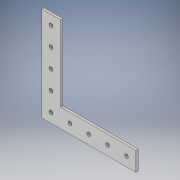
# Autodesk Inventor part: L gusset
Saved by Autodesk Inventor 2018 (Build 220112000, 112)
## iProperties
Created: 2019-01-13
Part Number: L gusset
Material: Generic
Document SubType Name: Modeling
Designer: s-2512711
Density: 1 g/cm^3
Appearance: Default
Author: s-2512711
Autodesk Inventor part; units mm, degrees
ref_plane "YZ Plane" through (0, 0, 0) normal (1, 0, 0) x (0, 1, 0)
ref_plane "XZ Plane" through (0, 0, 0) normal (0, 1, 0) x (-1, 0, 0)
ref_plane "XY Plane" through (0, 0, 0) normal (0, 0, 1) x (1, 0, 0)
sketch "Sketch1" plane through (0, 0, 0) normal (0, 0, 1) x (1, 0, 0)
  line L0 (0, 0) -> (76.2, 0)
  line L1 (76.2, 0) -> (76.2, 25.4)
  line L2 (76.2, 25.4) -> (25.4, 25.4)
  line L3 (0, 25.4) -> (0, 0)
  line L4 (0, 0) -> (25.4, 0)
  line L5 (25.4, 25.4) -> (25.4, 76.2)
  line L6 (25.4, 76.2) -> (0, 76.2)
  line L7 (0, 76.2) -> (0, 0)
  line L8 (12.7, 76.2) -> (12.7, 63.5) construction
  line L9 (12.7, 63.5) -> (12.7, 38.1) construction
  line L10 (12.7, 38.1) -> (12.7, 12.7) construction
  line L11 (12.7, 12.7) -> (38.1, 12.7) construction
  line L12 (38.1, 12.7) -> (63.5, 12.7) construction
  circle A0 centre (12.7, 63.5) radius 2.5797
  circle A1 centre (12.7, 38.1) radius 2.5797
  circle A2 centre (12.7, 12.7) radius 2.5797
  circle A3 centre (38.1, 12.7) radius 2.5797
  circle A4 centre (63.5, 12.7) radius 2.5797
  dimension "d0" = 76.2
  dimension "d1" = 25.4
  dimension "d2" = 25.4
  dimension "d3" = 76.2
  dimension "d4" = 12.7
  dimension "d5" = 25.4
  dimension "d6" = 25.4
  dimension "d7" = 25.4
  dimension "d8" = 25.4
  dimension "d9" = 5.1594
  constraints: 26 end point, 5 centre point, 5 coincident, 4 parallel, 3 perpendicular, 3 point on line, 2 horizontal, 1 midpoint, 1 vertical
  measures "d0" distance of L3.start L1.end
  measures "d1" distance of L1.end L0.end
  measures "d2" distance of L6.end L5.end
  measures "d3" distance of L5.end L4.end
  measures "d4" distance of L8.start L8.end
  measures "d5" distance of L8.end L9.end
  measures "d6" distance of L9.end L10.end
  measures "d7" distance of L10.end L11.end
  measures "d8" distance of L11.end L12.end
  measures "d9" diameter of A0
extrude "Extrusion1" add sketch "Sketch1" along normal blind 3.175
sketch "Sketch2" plane through (0, 0, 3.175) normal (0, 0, 1) x (1, 0, 0)
  circle A0 centre (12.7, 63.5) radius 2.5797 construction
  line L0 (12.7, 63.5) -> (12.7, 88.9) construction
  line L1 (12.7, 88.9) -> (12.7, 114.3) construction
  circle A1 centre (63.5, 12.7) radius 2.5797 construction
  line L2 (63.5, 12.7) -> (88.9, 12.7) construction
  line L3 (88.9, 12.7) -> (114.3, 12.7) construction
  circle A2 centre (88.9, 12.7) radius 2.5797
  circle A3 centre (114.3, 12.7) radius 2.5797
  circle A4 centre (12.7, 88.9) radius 2.5797
  circle A5 centre (12.7, 114.3) radius 2.5797
  line L4 (0, 76.2) -> (0, 0) projected
  line L5 (0, 76.2) -> (0, 127)
  line L6 (0, 127) -> (25.4, 127)
  line L7 (25.4, 25.4) -> (25.4, 76.2) projected
  line L8 (25.4, 127) -> (25.4, 76.2)
  line L9 (25.4, 76.2) -> (0, 76.2)
  line L10 (76.2, 0) -> (76.2, 25.4) projected
  line L11 (76.2, 25.4) -> (76.2, 0)
  line L12 (76.2, 0) -> (127, 0)
  line L13 (127, 0) -> (127, 25.4)
  line L14 (127, 25.4) -> (76.2, 25.4)
  dimension "d12" = 25.4
  dimension "d13" = 25.4
  dimension "d14" = 25.4
  dimension "d15" = 25.4
  dimension "d16" = 50.8
  dimension "d17" = 25.4
  dimension "d18" = 50.8
  constraints: 24 end point, 4 centre point, 4 coincident, 4 perpendicular, 3 vertical, 2 point on line, 1 horizontal
  measures "d12" distance of L0.start L0.end
  measures "d13" distance of L0.end L1.end
  measures "d14" distance of L2.start L2.end
  measures "d15" distance of L2.end L3.end
  measures "d16" distance of L4.start L5.end
  measures "d17" distance of L5.end L6.end
  measures "d18" distance of L10.start L12.end
extrude "Extrusion2" add sketch "Sketch2" against normal blind 3.175
body "Solid1"
